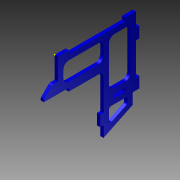
# Autodesk Inventor part: OpenROV 2_3 Dev Ducting Brace Mount
Saved by Autodesk Inventor 2012 (Build 160160000, 160)
## iProperties
Created: 2011-11-04
Part Number: OpenROV 2_3 Dev Ducting Brace Mount
Document SubType Name: Modeling
Designer: user
Density: 1 g/cm^3
Material: Default
Author: user
Autodesk Inventor part; units mm, degrees
ref_plane "YZ Plane" through (0, 0, 0) normal (1, 0, 0) x (0, 1, 0)
ref_plane "XZ Plane" through (0, 0, 0) normal (0, 1, 0) x (-1, 0, 0)
ref_plane "XY Plane" through (0, 0, 0) normal (0, 0, 1) x (1, 0, 0)
sketch "Sketch1" plane through (0, 0, 0) normal (0, 0, 1) x (1, 0, 0)
  point P0 (0, 0)
sketch "Sketch2" plane through (0, 0, 0) normal (1, 0, 0) x (0, 1, 0)
  line L0 (0, 0) -> (-20, 0)
  line L1 (-20, 0) -> (-20, 4.1716)
  line L2 (-23.1803, 0.4176) -> (-23.1803, 0.4176)
  line L3 (-23, -75) -> (-13, -75)
  line L4 (-13, -75) -> (-13, -72)
  line L5 (-13, -72) -> (0, -72)
  line L6 (0, -72) -> (0, -62)
  line L7 (0, -62) -> (-3, -62)
  line L8 (-3, -62) -> (-3, -10)
  line L9 (-3, -10) -> (0, -10)
  line L10 (0, -10) -> (0, 0)
  line L11 (-13, -5) -> (-20, -5)
  line L12 (-25, -10) -> (-25, -37)
  line L13 (-20, -42) -> (-13, -42)
  line L14 (-8, -37) -> (-8, -10)
  arc A0 (-8, -10) -> (-13, -5) centre (-13, -10) ccw
  arc A1 (-13, -42) -> (-8, -37) centre (-13, -37) ccw
  arc A2 (-25, -37) -> (-20, -42) centre (-20, -37) ccw
  arc A3 (-20, -5) -> (-25, -10) centre (-20, -10) ccw
  line L15 (-23, -72) -> (-23, -75)
  line L16 (-63, -69) -> (-63, -75)
  line L17 (-63, -75) -> (-53, -75)
  line L18 (-53, -75) -> (-53, -72)
  line L19 (-23, -72) -> (-53, -72)
  line L20 (-63, -69) -> (-73, -69)
  line L21 (-73, -69) -> (-86, -42)
  line L22 (-76, -42) -> (-76, -39)
  line L23 (-76, -39) -> (-66, -39)
  line L24 (-66, -39) -> (-66, -42)
  line L25 (-86, -42) -> (-76, -42)
  line L26 (-66, -42) -> (-38, -42)
  line L27 (-13, -47) -> (-46, -47)
  line L28 (-51, -52) -> (-51, -62)
  line L29 (-46, -67) -> (-13, -67)
  line L30 (-8, -62) -> (-8, -52)
  line L31 (-56, -52) -> (-59, -52)
  line L32 (-59, -52) -> (-59, -62)
  line L33 (-59, -62) -> (-56, -62)
  line L34 (-56, -62) -> (-56, -52)
  arc A4 (-8, -52) -> (-13, -47) centre (-13, -52) ccw
  arc A5 (-13, -67) -> (-8, -62) centre (-13, -62) ccw
  arc A6 (-51, -62) -> (-46, -67) centre (-46, -62) ccw
  arc A7 (-46, -47) -> (-51, -52) centre (-46, -52) ccw
  arc A8 (-38, -42) -> (-33, -37) centre (-38, -37) ccw
  line L35 (-33, -10) -> (-33, -37)
  line L36 (-30, 13) -> (-28.8284, 13)
  line L37 (-27.4142, 12.4142) -> (-20.5858, 5.5858)
  arc A9 (-27.4142, 12.4142) -> (-28.8284, 13) centre (-28.8284, 11) ccw
  arc A10 (-20, 4.1716) -> (-20.5858, 5.5858) centre (-22, 4.1716) ccw
  line L38 (-66, -47) -> (-74.8605, -47)
  line L39 (-76.6625, -49.8676) -> (-70.4032, -62.8676)
  line L40 (-68.6012, -64) -> (-66, -64)
  line L41 (-64, -62) -> (-64, -49)
  arc A11 (-70.4032, -62.8676) -> (-68.6012, -64) centre (-68.6012, -62) ccw
  arc A12 (-66, -64) -> (-64, -62) centre (-66, -62) ccw
  arc A13 (-64, -49) -> (-66, -47) centre (-66, -49) ccw
  arc A14 (-74.8605, -47) -> (-76.6625, -49.8676) centre (-74.8605, -49) ccw
  line L42 (-30, 13) -> (-30, -10)
  line L43 (-30, -10) -> (-33, -10)
  point P0 (-20, 5)
  point P1 (-25, -42)
  point P2 (-25, -5)
  point P3 (-30, -42)
  point P4 (-28, 13)
  dimension "d4" = 10
  dimension "d5" = 52
  dimension "d6" = 10
  dimension "d8" = 10
  dimension "d11" = 3
  dimension "d15" = 3
  dimension "d29" = 10
  dimension "d33" = 5
  dimension "d36" = 5
  dimension "d40" = 5
  dimension "d48" = 10
  dimension "d55" = 10
  dimension "d57" = 3
  dimension "d59" = 5
  dimension "d60" = 5
  dimension "d61" = 5
  dimension "d62" = 10
  dimension "d63" = 3
  dimension "d64" = 10
  dimension "d67" = 53
  dimension "d68" = 27
  dimension "d69" = 5
  dimension "d75" = 90
  dimension "d76" = 90
  dimension "d77" = 90
  dimension "d78" = 3
  dimension "d79" = 90
  dimension "d80" = 6
  dimension "d81" = 30
  dimension "d82" = 27
  dimension "d83" = 10
  dimension "d84" = 10
  dimension "d85" = 3
  dimension "d86" = 3
  dimension "d87" = 30
  dimension "d90" = 5
  dimension "d91" = 13
  dimension "d92" = 33
  dimension "d95" = 2
  dimension "d97" = 5
  dimension "d98" = 5
  dimension "d99" = 5
  dimension "d100" = 5
  dimension "d101" = 2
  dimension "d104" = 5
  dimension "d105" = 5
  dimension "d106" = 8
  dimension "d107" = 33
  dimension "d108" = 23
  dimension "d109" = 3
  dimension "d110" = 2
  dimension "d111" = 10
  constraints: 88 end point, 30 point on circle, 30 tangent, 20 parallel, 15 centre point, 11 equal radius, 9 perpendicular, 9 point on line, 6 horizontal
  measures "d4" distance of L9.end L0.start
  measures "d5" distance of L7.end L8.end
  measures "d6" distance of L5.end L6.end
  measures "d8" distance of L3.start L3.end
  measures "d11" distance of L8.end L9.end
  measures "d15" distance between parallel lines of L8 L6
  measures "d29" distance between parallel lines of L4 L8
  measures "d33" distance between parallel lines of L0 L11
  measures "d36" distance between parallel lines of L14 L8
  measures "d40" radius of A0
  measures "d48" distance of L16.end L17.end
  measures "d55" distance of L22.end L23.end
  measures "d57" distance of L23.end L24.end
  measures "d59" distance between parallel lines of L27 L26
  measures "d60" distance between parallel lines of L19 L29
  measures "d61" distance between parallel lines of L8 L30
  measures "d62" distance of L31.end L32.end
  measures "d63" distance of L32.end L33.end
  measures "d64" distance between parallel lines of L26 L31
  measures "d67" distance between parallel lines of L8 L34
  measures "d68" distance from line of L8 point (-30, -42)
  measures "d69" radius of A4
  measures "d75" angle of L19 L18
  measures "d76" angle of L19 L15
  measures "d77" angle of L16 L17
  measures "d78" distance between parallel lines of L19 L3
  measures "d79" angle of L24 L23
  measures "d80" distance of L16.start L16.end
  measures "d81" distance between parallel lines of L26 L19
  measures "d82" distance between parallel lines of L26 L20
  measures "d83" distance from line of L20.end L16
  measures "d84" distance from line of L21.end L22
  measures "d85" distance of L22.start L22.end
  measures "d86" distance of L3.end L4.end
  measures "d87" distance of L15.start L18.end
  measures "d90" distance of L0.end point (-20, 5)
  measures "d91" distance from line of L0 L36.start
  measures "d92" distance between parallel lines of L35 L10
  measures "d95" radius of A9
  measures "d97" distance between parallel lines of L39 L21
  measures "d98" distance between parallel lines of L26 L38
  measures "d99" distance between parallel lines of L41 L32
  measures "d100" distance between parallel lines of L20 L40
  measures "d101" radius of A11
  measures "d104" distance between parallel lines of L34 L28
  measures "d105" distance between parallel lines of L27 L13
  measures "d106" distance between parallel lines of L35 L12
  measures "d107" distance between parallel lines of L35 L24
  measures "d108" distance of L36.start L42.end
  measures "d109" distance of L42.end L35.start
  measures "d110" distance from line of point (-28, 13) L42
  measures "d111" distance between parallel lines of L1 L42
extrude "Extrusion5" add sketch "Sketch2" along normal blind 3
body "Solid5"
